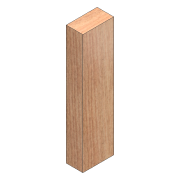
# Autodesk Inventor part: frameDepth
Saved by Autodesk Inventor 2018 (Build 220112000, 112)
## iProperties
Created: 2018-01-02
Part Number: frameDepth
Material: Wood (Birch)
Document SubType Name: Modeling
Designer: sawaiz
Density: 0.55 g/cm^3
Appearance: Birch - Natural Polished
Author: sawaiz
Autodesk Inventor part; units mm, degrees
ref_plane "YZ Plane" through (0, 0, 0) normal (1, 0, 0) x (0, 1, 0)
ref_plane "XZ Plane" through (0, 0, 0) normal (0, 1, 0) x (-1, 0, 0)
ref_plane "XY Plane" through (0, 0, 0) normal (0, 0, 1) x (1, 0, 0)
sketch "Sketch1" plane through (0, 0, 0) normal (0, 0, 1) x (1, 0, 0)
  line L0 (29, -54) -> (-29, -54)
  line L1 (-29, -54) -> (-29, 54)
  line L2 (-29, 54) -> (29, 54)
  line L3 (29, 54) -> (29, -54)
  line L4 (29, -54) -> (-29, 54) construction
  line L5 (-29, -54) -> (29, 54) construction
  point P0 (0, 0)
  dimension "d0" = 58
  dimension "d1" = 108
  constraints: 12 end point, 2 midpoint, 2 parallel, 1 horizontal, 1 perpendicular
  measures "d0" distance of L1.end L2.end
  measures "d1" distance of L0.end L1.end
extrude "Extrusion1" add sketch "Sketch1" along normal blind 419
equation "\"d0\" = lumberWidth"
equation "\"d1\" = lumberDepth"
equation "\"d2\" = -2 * frameOverhang + counterDepth - 2 * lumberWidth"
equation "\"lumberWidth\" = 58"
equation "\"lumberDepth\" = 108"
equation "\"counterThickness\" = 38"
equation "\"counterHeight\" = 858"
equation "\"counterDepth\" = 635"
equation "\"frameOverhang\" = 50"
body "Solid1"
